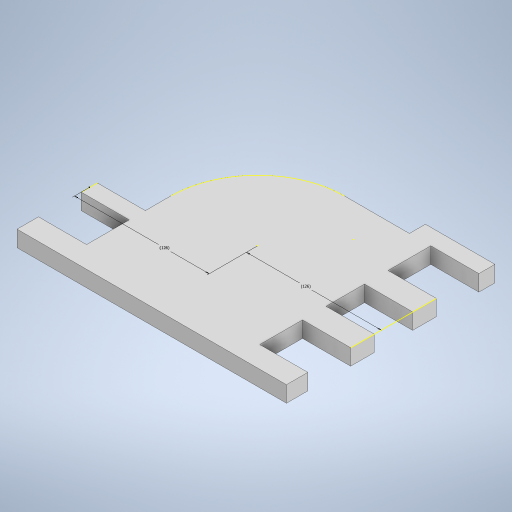
# Autodesk Inventor part: Zplita
Saved by Autodesk Inventor 2024 (Build 280153000, 153)
## iProperties
Created: 2023-11-12
Part Number: Zplita
Material: Generic
Document SubType Name: Modeling
Designer: KirikDK
Density: 1 g/cm^3
Appearance: Default
Author: KirikDK
Autodesk Inventor part; units mm, degrees
ref_plane "YZ Plane" through (0, 0, 0) normal (1, 0, 0) x (0, 1, 0)
ref_plane "XZ Plane" through (0, 0, 0) normal (0, 1, 0) x (-1, 0, 0)
ref_plane "XY Plane" through (0, 0, 0) normal (0, 0, 1) x (1, 0, 0)
sketch "Sketch1" plane through (0, 0, 0) normal (0, 1, 0) x (-1, 0, 0)
  line L0 (121, 129) -> (-41, 129)
  line L1 (-41, 129) -> (-41, -31)
  line L2 (-41, -31) -> (121, -31)
  line L3 (121, -31) -> (121, 129)
  line L4 (-86, 89) -> (166, 89)
  line L5 (166, 89) -> (166, 9)
  line L6 (166, 9) -> (-86, 9)
  line L7 (-86, 9) -> (-86, 89)
  line L8 (-86, 129) -> (166, 129)
  line L9 (166, 129) -> (166, 149)
  line L10 (166, 149) -> (-86, 149)
  line L11 (-86, 149) -> (-86, 129)
  line L12 (-21, -31) -> (-86, -31)
  line L13 (-86, -31) -> (-86, -46)
  line L14 (-86, -46) -> (-21, -46)
  line L15 (-21, -46) -> (-21, -31)
  line L16 (166, 9) -> (121, 9)
  line L17 (121, 9) -> (121, 74)
  line L18 (121, 74) -> (166, 74)
  line L19 (166, 74) -> (166, 9)
  point P0 (0, 0)
  point P1 (166, 139)
  point P2 (-86, -38.5)
  point P3 (121, 89)
  point P4 (121, 129)
  point P5 (-41, 89)
  point P6 (-41, 9)
  dimension "d0" = 162
  dimension "d1" = 160
  dimension "d2" = 40
  dimension "d5" = 40
  dimension "d7" = 45
  dimension "d8" = 45
  dimension "d9" = 20
  dimension "d10" = 45
  dimension "d11" = 15
  dimension "d12" = 45
  dimension "d13" = 20
  dimension "d14" = 15
  dimension "d32" = 0
  dimension "d33" = 45
  constraints: 40 end point, 10 parallel, 5 horizontal, 5 perpendicular, 2 midpoint, 2 point on line
  measures "d0" distance of L0.start L0.end
  measures "d1" distance of L0.end L1.end
  measures "d2" distance between parallel lines of L0 L4
  measures "d5" distance between parallel lines of L2 L6
  measures "d7" distance between parallel lines of L1 L7
  measures "d8" distance between parallel lines of L3 L5
  measures "d9" distance between parallel lines of L8 L10
  measures "d10" distance from line of L3 point (166, 139)
  measures "d11" distance between parallel lines of L12 L14
  measures "d12" distance from line of L1 point (-86, -38.5)
  measures "d13" distance between parallel lines of L1 L15
  measures "d14" distance between parallel lines of L4 L18
  measures "d32" distance between parallel lines of L0 L8
  measures "d33" distance of L0.end L8.start
extrude "Extrusion1" add sketch "Sketch1" along normal blind 15 contours L3 L4 L1 L0 | L0 L8 L11 L10 L9 | L4 L5 L18 L3 | L3 L6 L1 L4 | L1 L6 L7 L4 | L6 L3 L2 L1 | L2 L15 L14 L13 L12
fillet "Fillet1" radius 81 1 edges at (-121, 7.5, -31)
sketch "Sketch3" plane through (0, 15, 0) normal (0, 1, 0) x (1, 0, 0)
  arc A0 (-40, 31) -> (-121, -50) centre (-40, -50) ccw projected
  line L0 (86, -89) -> (86, -9) projected
  line L1 (-166, -74) -> (-166, -89) projected
  point P0 (0, 0)
  point P1 (-166, -81.5)
  dimension "d23" = 126
  dimension "d24" = 126
  constraints: 1 midpoint
  measures "d23" distance from line of L0 A0.centre
  measures "d24" horizontal distance of point (-166, -81.5) A0.centre
sketch "Sketch4" plane through (0, 15, 0) normal (0, 1, 0) x (1, 0, 0)
  line L0 (86, -67) -> (41, -67)
  line L1 (41, -67) -> (41, -31)
  line L2 (41, -31) -> (86, -31)
  line L3 (86, -31) -> (86, -67)
  line L4 (41, -89) -> (86, -89) projected
  line L5 (86, -89) -> (86, -9) projected
  line L6 (86, -9) -> (41, -9) projected
  point P0 (0, 0)
  point P1 (86, -49)
  dimension "d25" = 36
  dimension "d26" = 22
  dimension "d27" = 0
  dimension "d28" = 0
  dimension "d29" = 22
  constraints: 8 end point, 2 parallel, 1 horizontal, 1 midpoint, 1 perpendicular
  measures "d25" distance between parallel lines of L2 L0
  measures "d26" distance between parallel lines of L4 L0
  measures "d27" distance from line of L4.start L1
  measures "d28" distance from line of L5 point (86, -49)
  measures "d29" distance between parallel lines of L6 L2
extrude "Extrusion3" cut sketch "Sketch4" against normal blind 15
body "Solid1"
